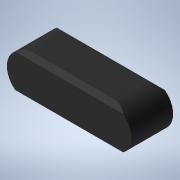
# Autodesk Inventor part: KESS2-6
Saved by Autodesk Inventor 2021 (Build 250183000, 183)
## iProperties
Created: 2025-02-08
Part Number: KESS2-6
Material: Generic
Catalog Web Link: www.cadenas.de
Description: KED, KEDH, KEDS, KES, KESH, KESS, KEG, KEGH, KEGS-Parallel Keys
Vendor: MISUMI
Document SubType Name: Modeling
Designer: psAdmin
Manufacturer: MISUMI
Mass: 0.0219104 g
Surface Area: 0.485643 cm^2
Volume: 0.0219104 cm^3
Density: 1 g/cm^3
Appearance: PSOLRGB-175-175-175
Category: PARTsolutions
Company: MISUMI
Title: KESS2-6
Author: Cadenas PARTsolutions
Comments: Parallel Keys
PSOL_IDENT_0: {$CADENAS_DATA/23d-libs/misumi/metric/28_keys_magnets/kegh.prj},214 {VTYP=3D},{NB=KESS2-6},{LINA=KES
PSOL_IDENT_1: S2-6},{NN=KED, KEDH, KEDS, KES, KESH, KESS, KEG, KEGH, KEGS},{DATE=29.11.2024 04:25:03},{GEOMDATE=22
PSOL_IDENT_2: .08.2013},{VERSION=},{LINEID=10},{WBVAR=TYS,MAT,HARD,L,ALT1,LC},{WBNUMERIC=L,LC}  {NB=KESS2-6},{LINA=
PSOL_IDENT_3: KESS2-6},{KT=DUMMY},{PN=KESS2-6},{PNALG=6},{TYS=KES},{TYPEALG='KEDS','KEDS','KESS','KESS','KEGS','KE
PSOL_IDENT_4: GS'},{MAT=S},{HARD=},{HARDALG='', '-'},{TS=600 or More},{B=2},{BTOL=0/-0.025},{L=6},{LALG=[6,8,10,15
PSOL_IDENT_5: ,20]},{LALG1=[0]},{ALT1=2},{LC=0},{LCALG=[0]},{LTOL=0},{H=2},{HTOL=0/-0.025},{C=0.16~0.25},{C1=0.200
PSOL_IDENT_6: },{CALG=[0.16:0.25/0.01]}
NB: KESS2-6
NN: KED, KEDH, KEDS, KES, KESH, KESS, KEG, KEGH, KEGS
NT: Parallel Keys
NBSYN: $PN.
LINA: KESS2-6
CATALOG: Misumi
PN: KESS2-6
TYS: Round
MAT: 316 Stainless Steel
HARD: -
TS: 600 or More
B: 2
BTOL: 0/-0.025
L: 6
ALT1: w/o LC (Changes Overall Length)
LC: 0
LTOL: 0
H: 2
HTOL: 0/-0.025
C: 0.16~0.25
SUPPLIER: MISUMI
ARTICLENO: KESS2-6
BOMINFO: KESS2-6
CREATOR: CADENAS GmbH
Autodesk Inventor part; units mm, degrees
ref_plane "YZ Plane" through (0, 0, 0) normal (1, 0, 0) x (0, 1, 0)
ref_plane "XZ Plane" through (0, 0, 0) normal (0, 1, 0) x (-1, 0, 0)
ref_plane "XY Plane" through (0, 0, 0) normal (0, 0, 1) x (1, 0, 0)
sketch "Sketch_7" plane through (0, 0, 0) normal (0, 0, 1) x (1, 0, 0)
  arc A0 (0, 1) -> (1, 0) centre (1, 1) ccw
  line L0 (1, 0) -> (5, 0)
  arc A1 (5, 0) -> (6, 1) centre (5, 1) ccw
  arc A2 (6, 1) -> (5, 2) centre (5, 1) ccw
  line L1 (5, 2) -> (1, 2)
  arc A3 (1, 2) -> (0, 1) centre (1, 1) ccw
  constraints: 8 point on circle, 4 centre point, 4 end point
extrude "Extrusion1" add sketch "Sketch_7" along normal blind 2
sketch "Sketch_8" plane through (0, 0, 0) normal (1, 0, 0) x (0, 1, 0)
  line L0 (-1, 3) -> (-1, -1)
  line L1 (-1, -1) -> (3, -1)
  line L2 (3, -1) -> (3, 3)
  line L3 (3, 3) -> (-1, 3)
  line L4 (1.8, 2) -> (0.2, 2)
  line L5 (0.2, 2) -> (0, 1.8)
  line L6 (0, 1.8) -> (0, 0.2)
  line L7 (0, 0.2) -> (0.2, 0)
  line L8 (0.2, 0) -> (1.8, 0)
  line L9 (1.8, 0) -> (2, 0.2)
  line L10 (2, 0.2) -> (2, 1.8)
  line L11 (2, 1.8) -> (1.8, 2)
  constraints: 24 end point
extrude "Extrusion2" cut sketch "Sketch_8" along normal blind 6
body "Solid1"
